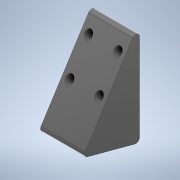
# Autodesk Inventor part: CC-bottomStand
Saved by Autodesk Inventor 2020 (Build 240168000, 168)
## iProperties
Created: 2019-07-03
Part Number: CC-bottomStand
Material: ABS Plastic
Document SubType Name: Modeling
Designer: andwh
Density: 1.06 g/cm^3
Appearance: Smooth - Black
Author: andwh
Autodesk Inventor part; units mm, degrees
ref_plane "YZ Plane" through (0, 0, 0) normal (1, 0, 0) x (0, 1, 0)
ref_plane "XZ Plane" through (0, 0, 0) normal (0, 1, 0) x (-1, 0, 0)
sketch "Sketch1" plane through (0, 0, 0) normal (1, 0, 0) x (0, 1, 0)
  line L0 (95.25, 0) -> (18.1319, 49.069)
  line L1 (0, 0) -> (0, -18.6) construction
  line L2 (95.25, 0) -> (4.9839, 0)
  line L3 (4.9839, 0) -> (18.1319, 49.069)
  dimension "d24" = 18.6
  dimension "d25" = 15
  dimension "d26" = 50.8
  dimension "d27" = 95.25
  constraints: 8 end point, 2 point on line, 1 horizontal, 1 vertical
  measures "d24" distance of L1.start L1.end
  measures "d25" angle of L1 L3
  measures "d26" distance of L2.end L0.end
  measures "d27" distance from line of L1 L0.start
extrude "Extrusion1" add sketch "Sketch1" along normal blind 38.1
fillet "Fillet1" radius 3.175 3 edges at (19.05, 95.25, 0) (19.05, 4.9839, 0) (19.05, 18.1319, 49.069)
ref_plane "Work Plane1" through (0, 20.0786, 47.2421) normal (0, 0, -1) x (-1, 0, 0)
sketch "Sketch2" plane through (0, 20.0786, 47.2421) normal (0, 0, -1) x (-1, 0, 0)
  line L0 (0, 65.9715) -> (0, 1.7044) projected
  line L1 (-38.1, -14.0238) -> (0, -14.0238) projected
  point P0 (0, -20.0786)
  point P1 (-6.35, 56.1214)
  point P2 (-6.35, 30.7214)
  point P3 (-31.75, 56.1214)
  point P4 (-31.75, 30.7214)
  dimension "d28" = 76.2
  dimension "d29" = 6.35
  dimension "d32" = 25.4
  dimension "d35" = 25.4
  constraints: 1 horizontal, 1 vertical, 3 other
  measures "d28" vertical distance of point (0, -20.079) point (-6.35, 56.121)
  measures "d29" distance from line of L0 point (-6.35, 56.121)
  measures "d32" distance of point (-6.35, 56.121) point (-6.35, 30.721)
  measures "d35" distance of point (-6.35, 56.121) point (-31.75, 56.121)
hole "Hole1" at (6.35, 76.2, 47.2421) at (31.75, 76.2, 47.2421) at (6.35, 50.8, 47.2421) at (31.75, 50.8, 47.2421) direction (0, 0, -1) diameter 3.4036 end through all counterbore diameter 6.2992 counterbore depth 44.45 clearance for "Flat Head Machine Screw" size "M3" standard "Ansi Metric M Profile"
body "Solid1"
